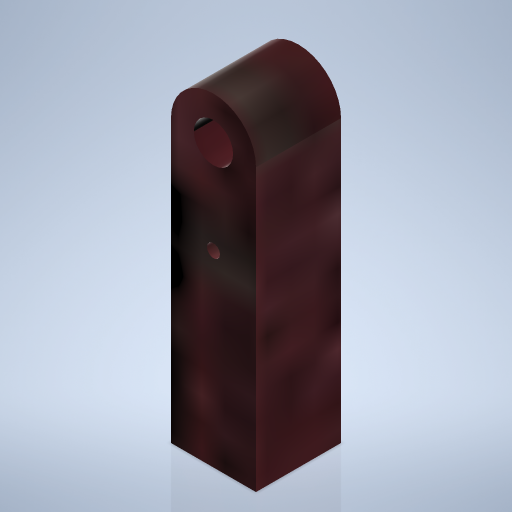
# Autodesk Inventor part: adapter
Saved by Autodesk Inventor 2024 (Build 280153000, 153)
## iProperties
Created: 2024-06-06
Part Number: adapter
Material: Aluminium 6061
Document SubType Name: Modeling
Designer: ffogue
Density: 2.7 g/cm^3
Appearance: 12 Zoll - Läuferverband - Burgund
Author: ffogue
Autodesk Inventor part; units mm, degrees
ref_plane "YZ Plane" through (0, 0, 0) normal (1, 0, 0) x (0, 1, 0)
ref_plane "XZ Plane" through (0, 0, 0) normal (0, 1, 0) x (-1, 0, 0)
ref_plane "XY Plane" through (0, 0, 0) normal (0, 0, 1) x (1, 0, 0)
sketch "Skizze1" plane through (0, 0, 0) normal (0, 1, 0) x (-1, 0, 0)
  line L0 (6.5, 0) -> (-6.5, 0)
  line L1 (-6.5, 0) -> (-6.5, 43)
  arc A0 (6.5, 43) -> (-6.5, 43) centre (0, 43) ccw
  line L2 (6.5, 43) -> (6.5, 0)
  line L3 (0, 0) -> (0, 43) construction
  point P0 (0, 0)
  dimension "d0" = 13
  dimension "d1" = 43
  dimension "d2" = 6.5
  dimension "d3" = 6.5
  constraints: 8 end point, 2 horizontal alignment, 2 point on circle, 1 centre point, 1 horizontal, 1 midpoint, 1 parallel, 1 perpendicular, 1 tangent, 1 vertical, 1 vertical alignment
  measures "d0" distance between parallel lines of L1 L2
  measures "d1" distance from line of L0 L3.end
  measures "d2" radius of A0
  measures "d3" distance of L0.end point (0, 0)
extrude "Extrusion1" add sketch "Skizze1" along normal blind 13
sketch "Skizze2" plane through (0, 13, 0) normal (0, 1, 0) x (1, 0, 0)
  arc A0 (-6.5, -43) -> (6.5, -43) centre (0, -43) ccw projected
  point P0 (0, 0)
  constraints: 1 coincident
hole "Bohrung1" at (0, 13, 43) direction (0, -1, 0) diameter 6 depth 13
sketch "Skizze3" plane through (6.5, 0, 0) normal (0, 0, -1) x (-1, 0, 0)
  circle A0 centre (6.5, 6.5) radius 3.5
  line L0 (0, 0) -> (0, 13) projected
  line L1 (0, 0) -> (13, 0) projected
  point P0 (6.5, 0)
  point P1 (0, 6.5)
  point P2 (6.5, 0)
  dimension "d13" = 7
  constraints: 2 midpoint, 1 centre point, 1 horizontal alignment, 1 vertical alignment
  measures "d13" diameter of A0
extrude "Extrusion2" cut sketch "Skizze3" against normal blind 36
sketch "Skizze4" plane through (0, 0, 0) normal (0, -1, 0) x (1, 0, 0)
  circle A0 centre (0, 43) radius 3 projected
  point P0 (0, 0)
  point P1 (0, 28.7)
  dimension "d23" = 14.3
  constraints: 1 vertical alignment
  measures "d23" distance of A0.centre point (0, 28.7)
hole "Bohrung2" at (0, 0, 28.7) direction (0, 1, 0) diameter 2 depth 4
